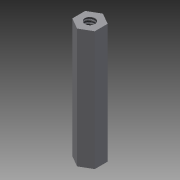
# Autodesk Inventor part: standoff
Saved by Autodesk Inventor 2015 (Build 190159000, 159)
## iProperties
Created: 2015-11-30
Part Number: standoff
Material: Generic
Document SubType Name: Modeling
Designer: jufranz
Density: 1 g/cm^3
Appearance: Default
Author: jufranz
Autodesk Inventor part; units mm, degrees
ref_plane "YZ Plane" through (0, 0, 0) normal (1, 0, 0) x (0, 1, 0)
ref_plane "XZ Plane" through (0, 0, 0) normal (0, 1, 0) x (-1, 0, 0)
ref_plane "XY Plane" through (0, 0, 0) normal (0, 0, 1) x (1, 0, 0)
sketch "Sketch1" plane through (0, 0, 0) normal (0, 1, 0) x (-1, 0, 0)
  line L0 (0, -2.7496) -> (-2.3812, -1.3748)
  line L1 (-2.3812, -1.3748) -> (-2.3813, 1.3748)
  line L2 (-2.3813, 1.3748) -> (0, 2.7496)
  line L3 (0, 2.7496) -> (2.3812, 1.3748)
  line L4 (2.3812, 1.3748) -> (2.3813, -1.3748)
  line L5 (2.3813, -1.3748) -> (0, -2.7496)
  point P0 (0, 0)
  point P1 (0, 0)
  dimension "d0" = 4.7625
  constraints: 12 end point, 1 coincident, 13 other
  measures "d0" distance between parallel lines of L1 L4
extrude "Extrusion1" add sketch "Sketch1" along normal blind 25.4
sketch "Sketch2" plane through (0, 25.4, 0) normal (0, 1, 0) x (1, 0, 0)
  point P0 (0, 0)
  point P1 (0, 0)
  constraints: 1 coincident
hole "Hole1" at (0, 25.4, 0) direction (0, -1, 0) diameter 2.159 end through all
body "Solid1"
